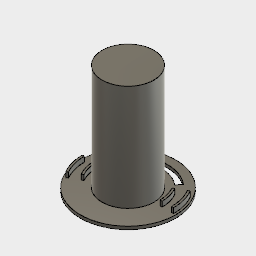
Gelatin_Mold_Top v5 (Autodesk Fusion 360 design; units mm, degrees)
Autodesk Fusion 360 part; units mm, degrees
sketch "Sketch1" plane through (0, 0, 0) normal (0, 1, 0) x (1, 0, 0)
  circle A0 centre (0, 0) radius 46
  dimension "d1" = 92
  measures "d1" diameter of A0
extrude "Extrude1" add sketch "Sketch1" along normal blind 3
sketch "Sketch2" plane through (0, 3, 0) normal (0, 1, 0) x (-1, 0, 0)
  circle A0 centre (0, 0) radius 46
  arc A1 (44, 0.0207) -> (38.1051, 22) centre (0, 0) ccw
  arc A2 (-44, 0.0207) -> (-38.1051, -22) centre (0, 0) ccw
  arc A3 (42, 0.0207) -> (36.3731, 21) centre (0, 0) ccw
  arc A4 (-42, 0.0207) -> (-36.3731, -21) centre (0, 0) ccw
  arc A5 (33, 0.0207) -> (28.5788, 16.5) centre (0, 0) ccw
  arc A6 (-33, 0.0207) -> (-28.5788, -16.5) centre (0, 0) ccw
  arc A7 (31, 0.0207) -> (26.8468, 15.5) centre (0, 0) ccw
  arc A8 (-31, 0.0207) -> (-26.8468, -15.5) centre (0, 0) ccw
  line L0 (-26.8468, -15.5) -> (-28.5788, -16.5)
  line L1 (-36.3731, -21) -> (-38.1051, -22)
  line L2 (-31, 0.0207) -> (-33, 0.0207)
  line L3 (-42, 0.0207) -> (-44, 0.0207)
  line L4 (0.0359, 0.0207) -> (0, 0)
  line L5 (44, 0.0207) -> (42, 0.0207)
  line L6 (33, 0.0207) -> (31, 0.0207)
  line L7 (38.1051, 22) -> (36.3731, 21)
  line L8 (28.5788, 16.5) -> (26.8468, 15.5)
  dimension "d8" = 30
  dimension "d9" = 30
  dimension "d23" = 42
  dimension "d24" = 44
  dimension "d25" = 42
  dimension "d26" = 33
  dimension "d27" = 31
  dimension "d28" = 31
  dimension "d29" = 33
  measures "d8" angle of L0 L5
  measures "d9" angle of L5 L7
  measures "d23" radius of A4
  measures "d24" radius of A2
  measures "d25" radius of A3
  measures "d26" radius of A6
  measures "d27" radius of A8
  measures "d28" radius of A7
  measures "d29" radius of A5
extrude "Extrude2" add sketch "Sketch2" along normal blind 5 contours A1 A3 L5 L7 | A2 A4 L1 L3 | A5 A7 L6 L8 | A6 A8 L0 L2
sketch "Sketch3" plane through (0, 3, 0) normal (0, 1, 0) x (-1, 0, 0)
  line L0 (44, 0.0207) -> (42, 0.0207)
  arc A0 (42, 0.0207) -> (36.3731, 21) centre (0, 0) ccw
  line L1 (36.3731, 21) -> (38.1051, 22)
  arc A1 (44, 0.0207) -> (38.1051, 22) centre (0, 0) ccw
  line L2 (-36.3731, -21) -> (-38.1051, -22)
  arc A2 (-44, 0.0207) -> (-38.1051, -22) centre (0, 0) ccw
  line L3 (-44, 0.0207) -> (-42, 0.0207)
  arc A3 (-42, 0.0207) -> (-36.3731, -21) centre (0, 0) ccw
  line L4 (33, 0.0207) -> (31, 0.0207)
  arc A4 (31, 0.0207) -> (26.8468, 15.5) centre (0, 0) ccw
  line L5 (26.8468, 15.5) -> (28.5788, 16.5)
  arc A5 (33, 0.0207) -> (28.5788, 16.5) centre (0, 0) ccw
  line L6 (-26.8468, -15.5) -> (-28.5788, -16.5)
  arc A6 (-33, 0.0207) -> (-28.5788, -16.5) centre (0, 0) ccw
  line L7 (-33, 0.0207) -> (-31, 0.0207)
  arc A7 (-31, 0.0207) -> (-26.8468, -15.5) centre (0, 0) ccw
  circle A8 centre (0, 0) radius 46
  line L8 (-20.4739, -24.5931) -> (-24.3128, -29.2043)
  line L9 (25.5175, -19.3096) -> (30.7614, -22.31)
  arc A9 (-24.3128, -29.2043) -> (30.7614, -22.31) centre (0, 0) ccw
  arc A10 (-20.4739, -24.5931) -> (25.5175, -19.3096) centre (0, 0) ccw
  arc A11 (28, 0.0207) -> (24.2487, 14) centre (0, 0) ccw
  arc A12 (-28, 0.0207) -> (-24.2487, -14) centre (0, 0) ccw
  dimension "d14" = 100
  dimension "d21" = 32
  dimension "d22" = 38
  measures "d14" angle of L8 L9
  measures "d21" radius of A10
  measures "d22" radius of A9
extrude "Extrude3" cut sketch "Sketch3" against normal blind 3 contours L8 L9 A9 A10
sketch "Sketch4" plane through (0, 3, 0) normal (0, 1, 0) x (-1, 0, 0)
  line L0 (25.5175, -19.3096) -> (30.7614, -22.31)
  arc A0 (-24.3128, -29.2043) -> (30.7614, -22.31) centre (0, 0) ccw
  line L1 (-24.3128, -29.2043) -> (-20.4739, -24.5931)
  arc A1 (-20.4739, -24.5931) -> (25.5175, -19.3096) centre (0, 0) ccw
  line L2 (44, 0.0207) -> (42, 0.0207)
  arc A2 (42, 0.0207) -> (36.3731, 21) centre (0, 0) ccw
  line L3 (36.3731, 21) -> (38.1051, 22)
  arc A3 (44, 0.0207) -> (38.1051, 22) centre (0, 0) ccw
  line L4 (-36.3731, -21) -> (-38.1051, -22)
  arc A4 (-44, 0.0207) -> (-38.1051, -22) centre (0, 0) ccw
  line L5 (-44, 0.0207) -> (-42, 0.0207)
  arc A5 (-42, 0.0207) -> (-36.3731, -21) centre (0, 0) ccw
  line L6 (33, 0.0207) -> (31, 0.0207)
  arc A6 (31, 0.0207) -> (26.8468, 15.5) centre (0, 0) ccw
  line L7 (26.8468, 15.5) -> (28.5788, 16.5)
  arc A7 (33, 0.0207) -> (28.5788, 16.5) centre (0, 0) ccw
  line L8 (-26.8468, -15.5) -> (-28.5788, -16.5)
  arc A8 (-33, 0.0207) -> (-28.5788, -16.5) centre (0, 0) ccw
  line L9 (-33, 0.0207) -> (-31, 0.0207)
  arc A9 (-31, 0.0207) -> (-26.8468, -15.5) centre (0, 0) ccw
  circle A10 centre (0, 0) radius 46
  circle A11 centre (0, 0) radius 25
  circle A12 centre (0, 0) radius 23
  dimension "d17" = 50
  dimension "d18" = 46
  measures "d17" diameter of A11
  measures "d18" diameter of A12
extrude "Extrude4" add sketch "Sketch4" along normal blind 102 contours A11
sketch "Sketch5" plane through (0, 105, 0) normal (0, 1, 0) x (-1, 0, 0)
  circle A0 centre (0, 0) radius 23
  circle A1 centre (0, 0) radius 25
  circle A2 centre (0, 0) radius 23
extrude "Extrude5" add sketch "Sketch5" against normal blind 2 contours A0 A2
